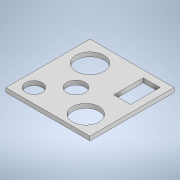
# Autodesk Inventor part: Holes_Test
Saved by Autodesk Inventor 2022 (Build 260153000, 153)
## iProperties
Created: 2021-07-13
Part Number: Holes_Test
Material: Generic
Document SubType Name: Modeling
Designer: MJAC
Density: 1 g/cm^3
Appearance: Default
Author: MJAC
Autodesk Inventor part; units mm, degrees
ref_plane "YZ Plane" through (0, 0, 0) normal (1, 0, 0) x (0, 1, 0)
ref_plane "XZ Plane" through (0, 0, 0) normal (0, 1, 0) x (-1, 0, 0)
ref_plane "XY Plane" through (0, 0, 0) normal (0, 0, 1) x (1, 0, 0)
sketch "Sketch1" plane through (0, 0, 0) normal (0, 1, 0) x (-1, 0, 0)
  line L0 (-30, -30) -> (30, -30)
  line L1 (30, -30) -> (30, 30)
  line L2 (30, 30) -> (-30, 30)
  line L3 (-30, 30) -> (-30, -30)
  line L4 (-30, -30) -> (30, 30) construction
  line L5 (30, -30) -> (-30, 30) construction
  point P0 (0, 0)
  dimension "d7" = 60
  dimension "d8" = 60
  constraints: 12 end point, 2 midpoint, 2 parallel, 1 horizontal, 1 perpendicular
  measures "d7" distance of L0.end L1.end
  measures "d8" distance of L1.end L2.end
extrude "Base plate" add sketch "Sketch1" along normal blind 3
sketch "Sketch2" plane through (0, 3, 0) normal (0, 1, 0) x (1, 0, 0)
  circle A0 centre (-5, -5) radius 6.5
  line L0 (-30, 30) -> (-30, -30) projected
  line L1 (-30, -30) -> (30, -30) projected
  point P0 (0, 0)
  dimension "d2" = 13
  dimension "d3" = 25
  dimension "d4" = 25
  constraints: 1 centre point
  measures "d2" diameter of A0
  measures "d3" distance from line of L0 A0.centre
  measures "d4" distance from line of L1 A0.centre
extrude "Tuimel" cut sketch "Sketch2" against normal through all
sketch "Sketch3" plane through (0, 3, 0) normal (0, 1, 0) x (1, 0, 0)
  circle A0 centre (-20, -20) radius 6
  line L0 (-30, 30) -> (-30, -30) projected
  line L1 (-30, -30) -> (30, -30) projected
  point P0 (0, 0)
  dimension "d9" = 12
  dimension "d10" = 10
  dimension "d11" = 10
  constraints: 1 centre point
  measures "d9" diameter of A0
  measures "d10" distance from line of L0 A0.centre
  measures "d11" distance from line of L1 A0.centre
extrude "Button" cut sketch "Sketch3" against normal through all
sketch "Sketch4" plane through (0, 3, 0) normal (0, 1, 0) x (1, 0, 0)
  circle A0 centre (-15, 15) radius 10
  line L0 (-30, 30) -> (-30, -30) projected
  line L1 (30, 30) -> (-30, 30) projected
  point P0 (0, 0)
  point P1 (-25, 0.0501)
  point P2 (-25, 19.9499)
  dimension "d14" = 20
  dimension "d15" = 15
  dimension "d16" = 15
  constraints: 1 centre point
  measures "d14" diameter of A0
  measures "d15" distance from line of L0 A0.centre
  measures "d16" distance from line of L1 A0.centre
extrude "Sleutel 20" cut sketch "Sketch4" against normal through all
sketch "Sketch5" plane through (0, 3, 0) normal (0, 1, 0) x (1, 0, 0)
  circle A0 centre (15, -18) radius 9.5
  line L0 (-30, 30) -> (-30, -30) projected
  line L1 (-30, -30) -> (30, -30) projected
  point P0 (0, 0)
  dimension "d19" = 19
  dimension "d20" = 45
  dimension "d21" = 12
  constraints: 1 centre point
  measures "d19" diameter of A0
  measures "d20" distance from line of L0 A0.centre
  measures "d21" distance from line of L1 A0.centre
extrude "Sleutel 19" cut sketch "Sketch5" against normal through all
sketch "Sketch6" plane through (0, 3, 0) normal (0, 1, 0) x (1, 0, 0)
  line L0 (13, 4) -> (25, 4)
  line L1 (25, 4) -> (25, 25)
  line L2 (25, 25) -> (13, 25)
  line L3 (13, 25) -> (13, 4)
  line L4 (13, 4) -> (25, 25) construction
  line L5 (25, 4) -> (13, 25) construction
  line L6 (30, 30) -> (-30, 30) projected
  line L7 (30, -30) -> (30, 30) projected
  point P0 (0, 0)
  point P1 (19, 14.5)
  dimension "d24" = 12
  dimension "d25" = 21
  dimension "d26" = 5
  dimension "d27" = 5
  constraints: 12 end point, 2 midpoint, 2 parallel, 1 horizontal, 1 perpendicular
  measures "d24" distance of L2.end L1.end
  measures "d25" distance of L1.end L0.end
  measures "d26" distance between parallel lines of L6 L2
  measures "d27" distance between parallel lines of L7 L1
extrude "Schakelaar" cut sketch "Sketch6" against normal through all
body "Solid1"
